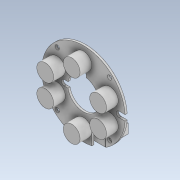
# Autodesk Inventor part: IRLed
Saved by Autodesk Inventor 2020 (Build 240168000, 168)
## iProperties
Created: 2021-07-14
Part Number: IRLed
Material: Generic
Document SubType Name: Modeling
Designer: Val
Density: 1 g/cm^3
Appearance: Default
Author: Val
Autodesk Inventor part; units mm, degrees
ref_plane "YZ Plane" through (0, 0, 0) normal (1, 0, 0) x (0, 1, 0)
ref_plane "XZ Plane" through (0, 0, 0) normal (0, 1, 0) x (-1, 0, 0)
ref_plane "XY Plane" through (0, 0, 0) normal (0, 0, 1) x (1, 0, 0)
sketch "Base" plane through (0, 0, 0) normal (0, 0, 1) x (1, 0, 0)
  circle A0 centre (0, 0) radius 22.35
  circle A1 centre (0, 0) radius 8.4
  dimension "d0" = 44.7
  dimension "d1" = 16.8
  constraints: 2 centre point, 2 coincident
  measures "d0" diameter of A0
  measures "d1" diameter of A1
extrude "BaseFeature" add sketch "Base" along normal blind 1.12
sketch "InsideProfile" plane through (0, 0, 1.12) normal (0, 0, 1) x (1, 0, 0)
  circle A0 centre (0, 0) radius 8.4 projected
  circle A1 centre (0, 0) radius 22.35 projected
  circle A2 centre (0, 0) radius 15.375 construction
  line L0 (0, 15.375) -> (0, -15.375) construction
  circle A3 centre (0, 15.375) radius 4.5
  circle A4 centre (0, -15.375) radius 4.5
  circle A5 centre (-14.1559, 6) radius 4.5
  circle A6 centre (-14.1559, -6) radius 4.5
  circle A7 centre (14.1559, 6) radius 4.5
  circle A8 centre (14.1559, -6) radius 4.5
  line L1 (0, 9.375) -> (0, 4.7505) construction
  line L2 (-1.5, 9.375) -> (-1.5, 4.7505)
  line L3 (1.5, 4.7505) -> (1.5, 9.375)
  arc A9 (1.5, 9.375) -> (-1.5, 9.375) centre (0, 9.375) ccw
  arc A10 (-1.5, 4.7505) -> (1.5, 4.7505) centre (0, 4.7505) ccw
  line L4 (0, -31.29) -> (0, 31.29) construction
  line L5 (-14.1559, 6) -> (-14.1559, -6) construction
  line L6 (-38.1332, 0) -> (38.1332, 0) construction
  line L7 (-10.3152, 0) -> (8.4348, 0) construction
  line L8 (-10.3152, 1.5) -> (8.4348, 1.5)
  line L9 (8.4348, -1.5) -> (-10.3152, -1.5)
  arc A11 (-10.3152, 1.5) -> (-10.3152, -1.5) centre (-10.3152, 0) ccw
  arc A12 (8.4348, -1.5) -> (8.4348, 1.5) centre (8.4348, 0) ccw
  line L10 (-25.738, 0) -> (-19.1152, 0) construction
  line L11 (-25.738, -1.5) -> (-19.1152, -1.5)
  line L12 (-19.1152, 1.5) -> (-25.738, 1.5)
  arc A13 (-25.738, 1.5) -> (-25.738, -1.5) centre (-25.738, 0) ccw
  arc A14 (-19.1152, -1.5) -> (-19.1152, 1.5) centre (-19.1152, 0) ccw
  line L13 (25.738, -1.5) -> (19.1152, -1.5)
  line L14 (19.1152, 1.5) -> (25.738, 1.5)
  arc A15 (25.738, -1.5) -> (25.738, 1.5) centre (25.738, 0) ccw
  arc A16 (19.1152, 1.5) -> (19.1152, -1.5) centre (19.1152, 0) ccw
  point P0 (0, 7.0627)
  point P1 (-14.1559, 0)
  point P2 (-0.9402, 0)
  point P3 (-22.4266, 0)
  point P4 (1.5, 8.265)
  point P5 (-1.5, 8.265)
  dimension "d4" = 13.95
  dimension "d5" = 6.975
  dimension "d6" = 9
  dimension "d8" = 12
  dimension "d9" = 1.5
  dimension "d10" = 2.3123
  dimension "d11" = 9.375
  dimension "d12" = 10.3152
  dimension "d13" = 9.375
  dimension "d14" = 8.8
  dimension "d15" = 15.4228
  constraints: 32 end point, 20 point on circle, 15 centre point, 13 tangent, 8 symmetric about line, 5 equal radius, 5 point on line, 4 midpoint, 3 coincident, 3 collinear, 3 parallel, 2 vertical, 4 other
  measures "d4" radial gap between concentric circles of A0 A1
  measures "d5" radial gap between concentric circles of A0 A2
  measures "d6" diameter of A3
  measures "d8" distance of L5.end L5.start
  measures "d9" radius of A9
  measures "d10" distance of point (0, 7.063) L1.start
  measures "d11" distance of L1.start point (0, 0)
  measures "d12" distance of L7.start point (0, 0)
  measures "d13" distance of L7.end point (-0.94, 0)
  measures "d14" distance of L7.start L10.end
  measures "d15" distance of L7.start L10.start
extrude "CutsFeature" cut sketch "InsideProfile" against normal through all contours A0 L9 L8 | A0 L8 A12 L9 | L3 A10 L2 A0 | A0 L2 A9 L3 | A0 L9 A11 L8 | A1 L13 A16 L14 | A1 L14 A15 L13 | L12 A14 L11 A1 | A1 L11 A13 L12
extrude "LightsFeature" add sketch "InsideProfile" along normal blind 6.3 contours A3 | A4 | A5 | A6 | A7 | A8
sketch "MountHoles" plane through (0, 0, 1.12) normal (0, 0, 1) x (1, 0, 0)
  circle A0 centre (-14, 14.5616) radius 1.15
  circle A1 centre (14, 14.5616) radius 1.15
  line L0 (-14, 14.5616) -> (14, 14.5616) construction
  circle A2 centre (0, 0) radius 21.35 construction
  arc A3 (22.2996, 1.5) -> (-22.2996, 1.5) centre (0, 0) ccw construction
  line L1 (-31.2195, 0) -> (31.2195, 0) construction
  circle A4 centre (-14, -14.5616) radius 1.15
  circle A5 centre (14, -14.5616) radius 1.15
  dimension "d20" = 28
  dimension "d21" = 2.3
  dimension "d22" = 2.3
  dimension "d23" = 1
  constraints: 5 centre point, 2 end point, 2 symmetric about line, 2 tangent, 1 coincident, 1 horizontal, 2 other
  measures "d20" distance of L0.start L0.end
  measures "d21" diameter of A0
  measures "d22" diameter of A1
  measures "d23" radial gap between concentric circles of A3 A2
extrude "MountHolesFeature" cut sketch "MountHoles" against normal through all
sketch "Sketch4" plane through (0, 0, 1.12) normal (0, 0, 1) x (1, 0, 0)
  arc A0 (-22.2996, -1.5) -> (22.2996, -1.5) centre (0, 0) ccw projected
  line L0 (12, -18.8553) -> (12, -14.8923)
  line L1 (12, -14.8923) -> (4.5, -14.8923)
  line L2 (4.5, -14.8923) -> (4.5, -21.8923)
  line L3 (4.5, -21.8923) -> (12, -21.8923)
  line L4 (12, -21.8923) -> (12, -18.8553)
  circle A1 centre (0, -15.375) radius 4.5 projected
  circle A2 centre (14, -14.5616) radius 1.15 projected
  dimension "d26" = 2
  dimension "d27" = 7
  constraints: 10 end point, 4 perpendicular, 2 point on circle, 1 tangent, 1 vertical
  measures "d26" horizontal distance of A2.centre L0.end
  measures "d27" distance of L1.end L2.end
extrude "Extrusion5" cut sketch "Sketch4" against normal through all contours L2 L1 L0 A0
sketch "Sketch5" plane through (0, 0, 0) normal (0, 0, -1) x (-1, 0, 0)
  line L0 (-4.5, -14.8923) -> (-12, -14.8923) projected
  line L1 (-4.5, -14.8923) -> (-10.6227, -14.8923)
  line L2 (-10.6227, -14.8923) -> (-10.6227, -19.9633)
  line L3 (-10.6227, -19.9633) -> (-4.5, -19.9633)
  line L4 (-4.5, -19.9633) -> (-4.5, -14.8923)
  point P0 (0, 0)
  dimension "d30" = 5.071
  dimension "d31" = 6.1227
  constraints: 8 end point, 2 parallel, 1 horizontal, 1 perpendicular
  measures "d30" distance of L1.end L2.end
  measures "d31" distance of L2.end L3.end
extrude "Extrusion6" add sketch "Sketch5" along normal blind 12.22
equation "\"d5\" = 0.5 * d4"
equation "\"d13\" = d11"
body "Solid1"
